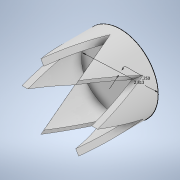
# Autodesk Inventor part: 3rd
Saved by Autodesk Inventor 2021 (Build 250183000, 183)
## iProperties
Created: 2020-07-12
Part Number: 3rd
Material: Generic
Document SubType Name: Modeling
Designer: saipr
Density: 1 g/cm^3
Appearance: Default
Author: saipr
Autodesk Inventor part; units mm, degrees
ref_plane "YZ Plane" through (0, 0, 0) normal (1, 0, 0) x (0, 1, 0)
ref_plane "XZ Plane" through (0, 0, 0) normal (0, 1, 0) x (-1, 0, 0)
ref_plane "XY Plane" through (0, 0, 0) normal (0, 0, 1) x (1, 0, 0)
sketch "Sketch1" plane through (0, 0, 0) normal (0, 0, 1) x (1, 0, 0)
  circle A0 centre (0, 0) radius 35.7251
  circle A1 centre (0, 0) radius 3.175
  dimension "d0" = 71.4502
  dimension "d3" = 6.35
  constraints: 2 centre point, 2 coincident
  measures "d0" diameter of A0
  measures "d3" diameter of A1
extrude "Extrusion1" add sketch "Sketch1" along normal blind 6.35
sketch "Sketch2" plane through (0, 0, 6.35) normal (0, 0, 1) x (1, 0, 0)
  line L0 (30.222182, 0) -> (30.222182, 19.05)
  circle A0 centre (0, 0) radius 35.7251
  line L1 (30.222182, 0) -> (30.222182, -19.05)
  arc A1 (30.222182, -19.05) -> (30.222182, 19.05) centre (0, 0) ccw
  line L2 (35.7251, 0) -> (30.222182, 0)
  line L3 (30.222182, 19.05) -> (24.719264, 19.05)
  line L4 (24.719264, 19.05) -> (24.719264, -19.05)
  line L5 (24.719264, -19.05) -> (30.222182, -19.05)
  arc A2 (24.719264, -19.05) -> (24.719264, 19.05) centre (-5.502918, 0) ccw
  dimension "d4" = 19.05
  dimension "d5" = 19.05
  dimension "d6" = 5.50292
  dimension "d7" = 5.50292
  constraints: 12 end point, 8 point on circle, 3 vertical, 2 centre point, 1 concentric, 1 horizontal, 1 perpendicular
  measures "d4" distance of L0.start L0.end
  measures "d5" distance of L0.start L1.end
  measures "d6" distance of L2.start L0.start
  measures "d7" distance of L0.end L3.end
extrude "Extrusion2" add sketch "Sketch2" along normal blind 50.8 contours A2 L3 L0 | L2 A0 L1 | L0 A0 L2 | L1 L5 A2
chamfer "Chamfer1" distance 50.8 angle 20.5505 1 edges at (27.4707, -19.05, 57.15) measured on face at (27.4707, -19.05, 56.65)
chamfer "Chamfer2" distance 50.8 angle 20.56 1 edges at (27.4707, 19.05, 57.15) measured on face at (27.4707, 19.05, 56.65)
pattern_circular "Circular Pattern2" count 6 over 360 about axis through (0, 0, 0) along (0, 0, 1) of "Extrusion2", "Chamfer1", "Chamfer2"
equation "\"d7\" = d6"
body "Solid1"
